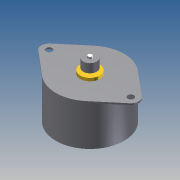
# Autodesk Inventor part: Stepper Motor SAIA 2012
Saved by Autodesk Inventor 2012 SP1 (Build 160190100, 190)
## iProperties
Shininess: 64.0
Length Units: 11269
Angle Units: 11279
Time Units: 11290
Mass Units: 11283
Length Display Precision: 3
Angle Display Precision: 2
Compacted: True
Part Number: Stepper Motor SAIA 2012
Document SubType Name: Modeling
Created: 2004-06-12
Designer: flg
Density: 1 g/cm^3
Material: Default
Density: 0.0
Volumn: 0.0
Area: 0.0
PropertySet Name: Model Information
Control State: 0
Master: False
Checked Out: False
Author: flg
Autodesk Inventor part; units mm, degrees
ref_plane "YZ Plane" through (0, 0, 0) normal (1, 0, 0) x (0, 1, 0)
ref_plane "XZ Plane" through (0, 0, 0) normal (0, 1, 0) x (-1, 0, 0)
ref_plane "XY Plane" through (0, 0, 0) normal (0, 0, 1) x (1, 0, 0)
sketch "Sketch1" plane through (0, 0, 0) normal (0, 0, 1) x (1, 0, 0)
  circle A0 centre (0, 0) radius 17.5
  dimension "d0" = 35
  constraints: 1 centre point
  measures "d0" diameter of A0
extrude "Extrusion1" add sketch "Sketch1" along normal blind 20.5
sketch "Sketch4" plane through (0, 0, 20.5) normal (0, 0, 1) x (1, 0, 0)
  arc A0 (17.5, 0) -> (17.5, 0) centre (0, 0) ccw projected
  circle A1 centre (0, 0) radius 5
  dimension "d15" = 10
  constraints: 1 centre point, 1 coincident, 1 concentric
  measures "d15" diameter of A1
extrude "Extrusion4" add sketch "Sketch4" along normal blind 2.3 contours A1
sketch "Sketch7" plane through (0, 0, 22.8) normal (0, 0, 1) x (1, 0, 0)
  circle A0 centre (0, 0) radius 5 projected
  circle A1 centre (0, 0) radius 1
  dimension "d24" = 2
  constraints: 1 centre point, 1 coincident, 1 concentric
  measures "d24" diameter of A1
extrude "Extrusion7" add sketch "Sketch7" along normal blind 6.5 contours A1
sketch "Sketch8" plane through (0, 0, 0) normal (0, 0, -1) x (-1, 0, 0)
  circle A0 centre (0, 0) radius 17.5 projected
  circle A1 centre (0, 0) radius 3
  dimension "d27" = 6
  constraints: 1 centre point, 1 coincident, 1 concentric
  measures "d27" diameter of A1
extrude "Extrusion8" add sketch "Sketch8" along normal blind 0.5 contours A1
sketch "Sketch9" plane through (0, 0, 20.5) normal (0, 0, 1) x (1, 0, 0)
  circle A0 centre (0, 0) radius 5 projected
  circle A1 centre (0, 0) radius 17.5 construction
  line L0 (-21, 0) -> (21, 0) construction
  line L1 (-25, 16.708) -> (-25, -1.9899) construction
  line L2 (-23.5714, -3.0639) -> (-11.25, -13.4048)
  line L3 (-23.5714, 3.0639) -> (-11.25, 13.4048)
  arc A2 (-23.5714, 3.0639) -> (-23.5714, -3.0639) centre (-21, 0) ccw
  arc A3 (23.5714, -3.0639) -> (23.5714, 3.0639) centre (21, 0) ccw
  line L4 (23.5714, 3.0639) -> (11.25, 13.4048)
  line L5 (23.5714, -3.0639) -> (11.25, -13.4048)
  arc A4 (-11.25, -13.4048) -> (11.25, -13.4048) centre (0, 0) ccw
  arc A5 (11.25, 13.4048) -> (-11.25, 13.4048) centre (0, 0) ccw
  dimension "d31" = 42
  dimension "d33" = 25
  constraints: 12 end point, 12 point on circle, 9 tangent, 4 centre point, 3 coincident, 2 midpoint, 1 equal radius, 1 horizontal, 1 perpendicular
  measures "d31" distance of L0.start L0.end
  measures "d33" distance from line of point (0, 0) L1
extrude "Extrusion9" add sketch "Sketch9" along normal blind 0.8
sketch "Sketch10" plane through (0, 0, 21.3) normal (0, 0, 1) x (1, 0, 0)
  circle A0 centre (0, 0) radius 5 construction
  arc A1 (-23.5714, 3.0639) -> (-23.5714, -3.0639) centre (-21, 0) ccw construction
  line L0 (-11.25, -13.4048) -> (-23.5714, -3.0639) construction
  arc A2 (-11.25, -13.4048) -> (11.25, -13.4048) centre (0, 0) ccw construction
  line L1 (23.5714, -3.0639) -> (11.25, -13.4048) construction
  arc A3 (23.5714, -3.0639) -> (23.5714, 3.0639) centre (21, 0) ccw construction
  line L2 (11.25, 13.4048) -> (23.5714, 3.0639) construction
  arc A4 (11.25, 13.4048) -> (-11.25, 13.4048) centre (0, 0) ccw construction
  line L3 (-23.5714, 3.0639) -> (-11.25, 13.4048) construction
  point P0 (0, 0)
hole "Hole1" at (-21, 0, 21.3) at (21, 0, 21.3) direction (0, 0, -1) diameter 3.15 end through all
sketch "Sketch11" plane through (0, 0, -0.5) normal (0, 0, -1) x (-1, 0, 0)
  circle A0 centre (0, 0) radius 1
  dimension "d43" = 2
  constraints: 1 centre point, 1 coincident
  measures "d43" diameter of A0
extrude "Extrusion10" add sketch "Sketch11" along normal blind 1
sketch "Sketch12" plane through (0, 0, 0) normal (1, 0, 0) x (0, 1, 0)
  line L0 (-1, 29.3) -> (1, 29.3) construction
  line L1 (-1, 22.8) -> (1, 22.8) construction
  line L2 (1, 28.3) -> (1, 23.8)
  line L3 (1, 23.8) -> (3.5, 23.8)
  line L4 (3.5, 23.8) -> (3.5, 28.3)
  line L5 (3.5, 28.3) -> (1, 28.3)
  line L6 (0, 29.3) -> (0, -6.1896) construction
  point P0 (0, 0)
  dimension "d47" = 1
  dimension "d48" = 4.5
  dimension "d49" = 7
  dimension "d50" = 2
  constraints: 10 end point, 3 perpendicular, 2 parallel, 1 midpoint
  measures "d47" distance from line of L3 L1.end
  measures "d48" distance of L3.end L4.end
  measures "d49" diameter of L4 L6
  measures "d50" diameter of L2 L6
revolve "Revolution1" add sketch "Sketch12" angle 360 about axis through (0, 0, 29.3) along (0, 0, -1)
body "Solid1"
